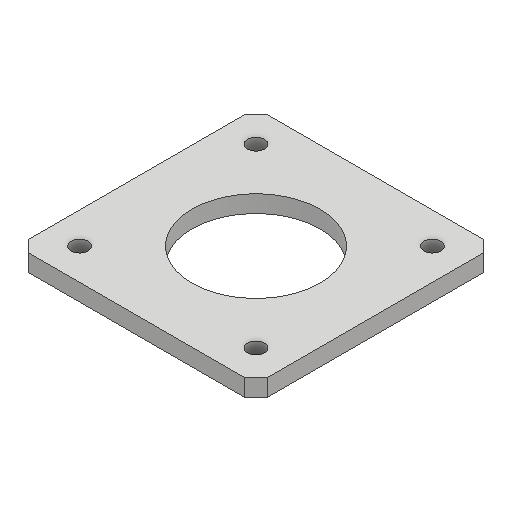
# Autodesk Inventor part: 3DP_ABS_X_Axis_Motor_Spacer
Saved by Autodesk Inventor 2026.1 (Build 301233000, 233)
## iProperties
Created: 2017-05-29
Part Number: 3DP_ABS_X_Axis_Motor_Spacer
Material: Ogólny
Document SubType Name: Modeling
Designer: Andrzej
Density: 1 g/cm^3
Appearance: Domyślna
Author: Andrzej
Autodesk Inventor part; units mm, degrees
ref_plane "YZ Plane" through (0, 0, 0) normal (1, 0, 0) x (0, 1, 0)
ref_plane "XZ Plane" through (0, 0, 0) normal (0, 1, 0) x (-1, 0, 0)
ref_plane "XY Plane" through (0, 0, 0) normal (0, 0, 1) x (1, 0, 0)
sketch "Szkic1" plane through (0, 0, 0) normal (0, 0, 1) x (1, 0, 0)
  line L0 (37.3233, -49.9659) -> (79.3233, -49.9659)
  line L1 (79.3233, -49.9659) -> (79.3233, -7.9659)
  line L2 (79.3233, -7.9659) -> (37.3233, -7.9659)
  line L3 (37.3233, -49.9659) -> (37.3233, -7.9659)
  point P0 (0, 0)
  point P1 (42.8233, -13.4659)
  point P2 (73.8233, -13.4659)
  point P3 (42.8233, -44.4659)
  point P4 (73.8233, -44.4659)
  point P5 (58.3233, -28.9659)
  dimension "d0" = 42
  dimension "d2" = 15.5
  dimension "d3" = 15.5
  dimension "d4" = 15.5
  dimension "d5" = 15.5
  dimension "d6" = 15.5
  dimension "d7" = 15.5
  dimension "d8" = 15.5
  dimension "d9" = 15.5
  dimension "d10" = 21
  dimension "d11" = 21
  dimension "d19" = 21
  constraints: 8 end point, 3 perpendicular, 1 horizontal
  measures "d0" distance between parallel lines of L0 L2
  measures "d2" horizontal distance of point (58.323, -28.966) point (42.823, -44.466)
  measures "d3" horizontal distance of point (58.323, -28.966) point (42.823, -44.466)
  measures "d4" horizontal distance of point (58.323, -28.966) point (42.823, -13.466)
  measures "d5" horizontal distance of point (58.323, -28.966) point (42.823, -13.466)
  measures "d6" horizontal distance of point (73.823, -13.466) point (58.323, -28.966)
  measures "d7" horizontal distance of point (58.323, -28.966) point (73.823, -13.466)
  measures "d8" horizontal distance of point (58.323, -28.966) point (73.823, -44.466)
  measures "d9" horizontal distance of point (58.323, -28.966) point (73.823, -44.466)
  measures "d10" distance from line of L2 point (58.323, -28.966)
  measures "d11" distance from line of L1 point (58.323, -28.966)
  measures "d19" distance from line of L3 point (58.323, -28.966)
extrude "Wyciągnięcie proste1" add sketch "Szkic1" along normal blind 3
hole "Otwór1" at (73.8233, -44.4659, 0) at (42.8233, -44.4659, 0) at (73.8233, -13.4659, 0) at (42.8233, -13.4659, 0) direction (0, 0, 1) diameter 3 end through all
hole "Otwór2" at (58.3233, -28.9659, 0) direction (0, 0, 1) diameter 22.5 end through all
chamfer "Faza1" distance 2 angle 45 4 edges at (37.3233, -7.9659, 1.5) (79.3233, -7.9659, 1.5) (79.3233, -49.9659, 1.5) (37.3233, -49.9659, 1.5)
equation "\"d2\" = 0.5 * d18"
equation "\"d3\" = d2"
equation "\"d4\" = d2"
equation "\"d11\" = d10"
equation "\"d18\" = 31"
